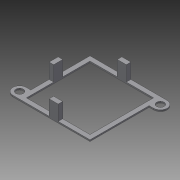
# Autodesk Inventor part: Stepper_Motor_Holder-SquareBar-Rev3
Saved by Autodesk Inventor 2015 (Build 190159000, 159)
## iProperties
Created: 2017-01-12
Part Number: Stepper_Motor_Holder-SquareBar-Rev3
Material: Generic
Document SubType Name: Modeling
Designer: Guy
Density: 1 g/cm^3
Appearance: Default
Mass: 1.16195 g
Surface Area: 21.9998 cm^2
Volume: 1.16195 cm^3
Author: Guy
Autodesk Inventor part; units mm, degrees
ref_plane "YZ Plane" through (0, 0, 0) normal (1, 0, 0) x (0, 1, 0)
ref_plane "XZ Plane" through (0, 0, 0) normal (0, 1, 0) x (-1, 0, 0)
ref_plane "XY Plane" through (0, 0, 0) normal (0, 0, 1) x (1, 0, 0)
sketch "Sketch1" plane through (0, 0, 0) normal (0, 0, 1) x (1, 0, 0)
  line L0 (0, 0) -> (42.3, 0)
  line L1 (42.3, 0) -> (42.3, 42.3)
  line L2 (42.3, 42.3) -> (0, 42.3)
  line L3 (0, 42.3) -> (0, 0)
  line L4 (45.3, -3) -> (45.3, 45.3)
  line L5 (-3, 45.3) -> (-3, -3)
  line L6 (-6, -3) -> (45.3, -3)
  line L7 (-3, 45.3) -> (48.3, 45.3)
  circle A0 centre (48.3, 40.8) radius 2.5
  arc A1 (48.3, 36.3) -> (48.3, 45.3) centre (48.3, 40.8) ccw
  line L8 (45.3, 36.3) -> (48.3, 36.3)
  circle A2 centre (-6, 1.5) radius 2.5
  arc A3 (-6, 6) -> (-6, -3) centre (-6, 1.5) ccw
  line L9 (-3, 6) -> (-6, 6)
  point P0 (45.3, 42.3)
  point P1 (45.3, 0)
  point P2 (-3, 0)
  point P3 (-3, 42.3)
  dimension "d0" = 42.3
  dimension "d1" = 42.3
  dimension "d3" = 3
  dimension "d5" = 3
  dimension "d29" = 3
  dimension "d43" = 3
  dimension "d50" = 5
  dimension "d51" = 9
  dimension "d52" = 3
  dimension "d61" = 5
  dimension "d62" = 9
  dimension "d63" = 3
  constraints: 20 end point, 8 point on line, 4 centre point, 4 horizontal, 4 point on circle, 4 tangent, 3 parallel, 2 coincident, 2 perpendicular
  measures "d0" distance of L0.end L1.end
  measures "d1" distance of L1.end L2.end
  measures "d3" distance between parallel lines of L4 L1
  measures "d5" distance between parallel lines of L3 L5
  measures "d29" distance between parallel lines of L6 L0
  measures "d43" distance between parallel lines of L2 L7
  measures "d50" diameter of A0
  measures "d51" diameter of A1
  measures "d52" distance from line of L4 A1.centre
  measures "d61" diameter of A2
  measures "d62" diameter of A3
  measures "d63" distance from line of L5 A2.centre
extrude "Extrusion7" add sketch "Sketch1" along normal blind 1
sketch "Sketch3" plane through (0, 0, 1) normal (0, 0, 1) x (1, 0, 0)
  line L0 (0, 0) -> (0, 42.3) projected
  line L1 (0, 42.3) -> (42.3, 42.3) projected
  line L2 (42.3, 42.3) -> (42.3, 0) projected
  line L3 (42.3, 0) -> (0, 0) projected
  circle A0 centre (48.3, 40.8) radius 2.5 projected
  circle A1 centre (-6, 1.5) radius 2.5 projected
  line L4 (-3, 6) -> (-6, 6) projected
  arc A2 (-6, 6) -> (-6, -3) centre (-6, 1.5) ccw projected
  line L5 (-6, -3) -> (45.3, -3) projected
  line L6 (45.3, -3) -> (45.3, 36.3) projected
  line L7 (45.3, 36.3) -> (48.3, 36.3) projected
  arc A3 (48.3, 36.3) -> (48.3, 45.3) centre (48.3, 40.8) ccw projected
  line L8 (48.3, 45.3) -> (-3, 45.3) projected
  line L9 (-3, 45.3) -> (-3, 6) projected
  line L10 (0, 42.3) -> (0, 0) projected
  line L11 (-3, 24.15) -> (0, 24.15)
  line L12 (0, 24.15) -> (0, 18.15)
  line L13 (0, 18.15) -> (-3, 18.15)
  line L14 (-3, 18.15) -> (-3, 24.15)
  line L15 (42.3, 24.15) -> (45.3, 24.15)
  line L16 (45.3, 24.15) -> (45.3, 18.15)
  line L17 (45.3, 18.15) -> (42.3, 18.15)
  line L18 (42.3, 18.15) -> (42.3, 24.15)
  line L19 (18.15, 45.3) -> (24.15, 45.3)
  line L20 (24.15, 45.3) -> (24.15, 42.3)
  line L21 (24.15, 42.3) -> (18.15, 42.3)
  line L22 (18.15, 42.3) -> (18.15, 45.3)
  line L23 (42.3, 0) -> (0, 0) projected
  line L24 (18.15, 0) -> (24.15, 0)
  line L25 (24.15, 0) -> (24.15, -3)
  line L26 (24.15, -3) -> (18.15, -3)
  line L27 (18.15, -3) -> (18.15, 0)
  dimension "d66" = 6
  dimension "d67" = 6
  dimension "d68" = 6
  dimension "d69" = 6
  dimension "d70" = 18.15
  dimension "d71" = 18.15
  dimension "d72" = 18.15
  constraints: 32 end point, 9 point on line, 8 parallel, 4 horizontal, 4 perpendicular
  measures "d66" distance between parallel lines of L20 L22
  measures "d67" distance between parallel lines of L17 L15
  measures "d68" distance between parallel lines of L27 L25
  measures "d69" distance between parallel lines of L13 L11
  measures "d70" distance between parallel lines of L10 L22
  measures "d71" distance between parallel lines of L0 L27
  measures "d72" distance between parallel lines of L1 L15
extrude "Extrusion9" add sketch "Sketch3" along normal blind 10 contours L13 L9 L11 L0 | L3 L25 L5 L27 | L22 L8 L20 L1
body "Solid6"
